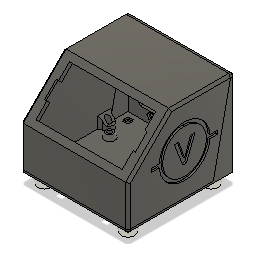
Voltímetro v10 (Autodesk Fusion 360 design; units mm, degrees)
Autodesk Fusion 360 part; units mm, degrees
note: some values were not read from the file. Set by a fixed rule: which face or edge a step refers to.
sketch "Sketch3" plane through (0, 0, 0) normal (0, 1, 0) x (1, 0, 0)
  circle A0 centre (-30.465, -17.5) radius 1.03 construction
  circle A1 centre (24.465, -17.5) radius 1.03 construction
  circle A2 centre (-30.465, 17.5) radius 1.03 construction
  circle A3 centre (24.465, 17.5) radius 1.03 construction
  line L0 (-30.465, 17.5) -> (24.465, 17.5) construction
  line L1 (24.465, 17.5) -> (24.465, -17.5) construction
  line L2 (24.465, -17.5) -> (-30.465, -17.5) construction
  line L3 (-30.465, -17.5) -> (-30.465, 17.5) construction
  line L4 (-30.465, 0) -> (24.465, 0) construction
  line L5 (-3, 17.5) -> (-3, -17.5) construction
  line L6 (-45, -42.5) -> (45, -42.5)
  line L7 (45, -42.5) -> (45, 47.5)
  line L8 (45, 47.5) -> (-45, 47.5)
  line L9 (-45, 47.5) -> (-45, -42.5)
  line L10 (0, -42.5) -> (0, 47.5) construction
  line L11 (-45, 44) -> (45, 44)
  circle A4 centre (-30.465, 17.5) radius 1.75
  circle A5 centre (-30.465, -17.5) radius 1.75
  circle A6 centre (24.465, -17.5) radius 1.75
  circle A7 centre (24.465, 17.5) radius 1.75
  circle A8 centre (-30.465, 17.5) radius 3.07
  circle A9 centre (-30.465, -17.5) radius 3.07
  circle A10 centre (24.465, -17.5) radius 3.07
  circle A11 centre (24.465, 17.5) radius 3.07
  dimension "d3" = 35
  dimension "d4" = 35
  dimension "d5" = 54.93
  dimension "d6" = 54.93
  dimension "d8" = 2.06
  dimension "d9" = 2.06
  dimension "d10" = 2.06
  dimension "d11" = 2.06
  dimension "d12" = 25
  dimension "d13" = 90
  dimension "d15" = 30
  dimension "d23" = 3.5
  dimension "d67" = 3.5
  dimension "d68" = 3.5
  dimension "d69" = 3.5
  dimension "d70" = 3.5
  dimension "d71" = 1.32
  dimension "d72" = 1.32
  dimension "d73" = 1.32
  dimension "d74" = 1.32
  dimension "d161" = 3
  constraint coincident A2.centre L0.start
  constraint coincident A3.centre L0.end
  constraint coincident A1.centre L1.end
  constraint coincident A0.centre L2.end
  constraint horizontal L0
  constraint vertical L3
  constraint midpoint L3 L4.start
  constraint midpoint L1 L4.end
  constraint midpoint L0 L5.start
  constraint midpoint L2 L5.end
  constraint horizontal L6
  constraint vertical L7
  constraint horizontal L8
  constraint vertical L9
  constraint midpoint L6 L10.start
  constraint midpoint L8 L10.end
  constraint coincident origin L10
  constraint coincident origin L4
  constraint coincident L9 L11.start
  constraint coincident L7 L11.end
  constraint perpendicular L7 L11
  constraint concentric A0 A5
  constraint concentric A1 A6
  constraint concentric A3 A7
  measures "d3" vertical distance of A0.centre A2.centre
  measures "d4" vertical distance of A1.centre A3.centre
  measures "d5" horizontal distance of A0.centre A1.centre
  measures "d6" horizontal distance of A2.centre A3.centre
  measures "d8" diameter of A2
  measures "d9" diameter of A3
  measures "d10" diameter of A1
  measures "d11" diameter of A0
  measures "d12" distance of L2 L6
  measures "d13" distance of L7 L9
  measures "d15" distance of L0 L8
  measures "d23" distance of L8 L11
  measures "d67" diameter of A4
  measures "d68" diameter of A5
  measures "d69" diameter of A6
  measures "d70" diameter of A7
  measures "d161" distance of L5 L10
extrude "Extrude1" add sketch "Sketch3" against normal blind 3.5 contours L6 L7 L9 L11 | L7 L8 L9 L11 | A4 | A5 | A6 | A7 | A8 | A9 | A10 | A11 makes body 1
sketch "Sketch4" plane through (0, 0, 0) normal (1, 0, 0) x (0, 0, -1)
  line L0 (-29.1643, 58.8035) -> (-68.5643, 58.8035)
  line L1 (-68.5643, 58.8035) -> (-68.5643, 33.8035)
  line L2 (-68.5643, 33.8035) -> (-29.1643, 33.8035)
  line L3 (-29.1643, 33.8035) -> (-29.1643, 58.8035)
  dimension "d19" = 25
  dimension "d20" = 39.4
  constraint horizontal L0
  constraint vertical L1
  constraint horizontal L2
  constraint vertical L3
  measures "d19" distance of L0 L2
  measures "d20" distance of L1 L3
extrude "Extrude2" add sketch "Sketch4" along normal mid plane 72 separate body makes body 2
move_body "Move1" bodies 2 to x (1, 0, 0) y (0, 0.707107, 0.707107) z (0, -0.707107, 0.707107) at (0, 49.8005, -24.0063)
extrude "Extrude3" add sketch "Sketch3" along normal blind 70 contours L7 L8 L9 L11 bodies 1
sketch "Sketch5" plane through (45, 0, 0) normal (1, 0, 0) x (0, 0, -1)
  line L0 (-42.5, 0) -> (47.5, 0)
  line L1 (44, 70) -> (29.121, 0)
  line L2 (44, 70) -> (135.3221, 70) construction
  line L3 (44, 0) -> (44, 70)
  point P0 (44, 70)
  dimension "d26" = 102
  constraint horizontal L2
  constraint coincident P0 L1.start
  constraint coincident L0 L1.end
  measures "d26" angle of L1 L2
extrude "Extrude4" add sketch "Sketch5" against normal blind 3.5 bodies 1
extrude "Extrude5" add sketch "Sketch5" along normal blind 3.5 from surface at -90 bodies 1
extrude "Extrude6" add sketch "Sketch3" along normal blind 70 separate body contours L6 L7 L9 L11 | L7 L8 L9 L11 | A4 | A5 | A6 | A7 | A8 | A9 | A10 | A11 makes body 3
chamfer "Chamfer1" distance 36 angle 45 1 edges at (0, 70, 42.5) on bodies 3
move_body "Move2" bodies 2 to x (1, 0, 0) y (0, 1, 0) z (0, 0, 1) at (0, 1.9818, -4.5415)
shell "Shell1" thickness 3.5 removed faces 1 at (-15, 0, 12.5) on bodies 3
combine "Combine1" operation cut target body 3 tool bodies 1 keep tools
sketch "Sketch6" plane through (0, 38.25, 38.25) normal (0, 0.707107, 0.707107) x (1, 0, 0)
  line L0 (45, -6.0104) -> (45, 44.9013)
  line L1 (45, 44.9013) -> (-45, 44.9013)
  line L2 (-45, 44.9013) -> (-45, -6.0104)
  line L3 (-45, -6.0104) -> (45, -6.0104)
  line L4 (-45, 19.4454) -> (45, 19.4454) construction
  line L5 (0, 44.9013) -> (0, -6.0104) construction
  line L6 (-36.2, 39.3454) -> (36.2, 39.3454)
  line L7 (36.2, 39.3454) -> (36.2, -0.4546)
  line L8 (36.2, -0.4546) -> (-36.2, -0.4546)
  line L9 (-36.2, -0.4546) -> (-36.2, 39.3454)
  line L10 (-36.2, 39.3454) -> (36.2, -0.4546) construction
  line L11 (36.2, 39.3454) -> (-36.2, -0.4546) construction
  point P0 (0, 19.4454)
  dimension "d151" = 2
  constraint midpoint L2 L4.start
  constraint midpoint L0 L4.end
  constraint midpoint L1 L5.start
  constraint midpoint L3 L5.end
  constraint horizontal L6
  constraint perpendicular L6 L7
  constraint parallel L6 L8
  constraint parallel L7 L9
  constraint coincident L10 P0
  constraint coincident L11 P0
  constraint midpoint L5 P0
  measures "d36" distance of L7.end L8.end
  measures "d37" distance of L6.end L7.end
extrude "Extrude7" cut sketch "Sketch6" against normal blind 10 contours L6 L7 L8 L9 bodies 3
sketch "Sketch7" plane through (0, 0, -47.5) normal (0, 0, -1) x (-1, 0, 0)
  line L0 (8.8, 56.65) -> (36, 56.65) construction
  line L1 (36, 56.65) -> (36, 15.1533) construction
  line L2 (30.6967, 9.85) -> (14.1033, 9.85) construction
  line L3 (8.8, 15.1533) -> (8.8, 56.65) construction
  line L4 (14.1033, 9.85) -> (8.8, 15.1533) construction
  line L5 (36, 15.1533) -> (30.6967, 9.85) construction
  line L6 (22.4, 56.65) -> (22.4, 9.85) construction
  line L7 (22.4, 33.25) -> (8.8, 33.25) construction
  circle A0 centre (22.4, 60.75) radius 1.75
  circle A1 centre (22.4, 5.75) radius 1.75
  line L8 (36.5, 57.15) -> (36.5, 14.9462)
  line L9 (36.5, 14.9462) -> (30.9038, 9.35)
  line L10 (30.9038, 9.35) -> (13.8962, 9.35)
  line L11 (13.8962, 9.35) -> (8.3, 14.9462)
  line L12 (8.3, 14.9462) -> (8.3, 57.15)
  line L13 (8.3, 57.15) -> (36.5, 57.15)
  line L14 (-45, 70) -> (-45, -3.5) construction
  line L15 (-45, -3.5) -> (45, -3.5) construction
  line L16 (45, -3.5) -> (45, 70) construction
  line L17 (45, 70) -> (-45, 70) construction
  line L18 (45, 33.25) -> (36.5, 33.25) construction
  line L19 (37.7, 58.35) -> (37.7, 14.4491) construction
  line L20 (37.7, 14.4491) -> (31.4009, 8.15) construction
  line L21 (31.4009, 8.15) -> (13.3991, 8.15) construction
  line L22 (13.3991, 8.15) -> (7.1, 14.4491) construction
  line L23 (7.1, 14.4491) -> (7.1, 58.35) construction
  line L24 (7.1, 58.35) -> (37.7, 58.35) construction
  point P0 (36, 9.85)
  point P1 (8.8, 9.85)
  dimension "d40" = 27.2
  dimension "d41" = 46.8
  dimension "d42" = 5.3033
  dimension "d43" = 5.3033
  dimension "d44" = 5.3033
  dimension "d45" = 5.3033
  dimension "d47" = 3.5
  dimension "d48" = 55
  dimension "d49" = -0.5
  dimension "d53" = 8.5
  dimension "d61" = -1.7
  constraint horizontal L0
  constraint vertical L1
  constraint horizontal L2
  constraint vertical L3
  constraint coincident P1 L2
  constraint coincident P1 L3
  constraint coincident P0 L1
  constraint coincident P0 L2
  constraint midpoint L0 L6.start
  constraint midpoint L2 L6.end
  constraint midpoint L6 L7.start
  constraint coincident L3 L7.end
  constraint perpendicular L3 L7
  constraint coincident L6 A0.centre
  constraint symmetric L7 A0 A1
  constraint midpoint L16 L18.start
  constraint perpendicular L16 L18
  constraint collinear L7 L18
  constraint coincident L8 L18.end
  measures "d40" distance of L0.start L0.end
  measures "d41" distance of L0.start P1
  measures "d42" distance of P1 L2.end
  measures "d43" distance of P1 L3.start
  measures "d44" distance of P0 L1.end
  measures "d45" distance of P0 L2.start
  measures "d47" diameter of A0
  measures "d48" distance of A0.centre A1.centre
  measures "d53" distance of L18.start L18.end
sketch "Sketch8" plane through (0, 0, -47.5) normal (0, 0, -1) x (-1, 0, 0)
  line L0 (-45, 70) -> (-45, -3.5)
  line L1 (-45, -3.5) -> (45, -3.5)
  line L2 (45, -3.5) -> (45, 70)
  line L3 (45, 70) -> (-45, 70)
  line L4 (-45, 33.25) -> (45, 33.25) construction
  circle A0 centre (-27.8532, 33.2847) radius 4.25
  line L5 (-27.8532, 33.2847) -> (-6.5468, 33.2847) construction
  circle A1 centre (-6.5468, 33.2847) radius 4.25
  line L6 (-17.2, 33.2847) -> (-17.2, 33.2153)
  circle A2 centre (-6.5468, 33.2847) radius 5 construction
  circle A3 centre (-27.8532, 33.2847) radius 5 construction
  line L7 (-41.5, 70) -> (-41.5, -3.5) construction
  line L8 (-45, 70) -> (-45, -3.5) construction
  line L9 (-27.8532, 33.2847) -> (-27.8532, 38.2847) construction
  line L10 (-27.8532, 38.2847) -> (-30.0921, 36.8972)
  line L11 (-27.8532, 38.2847) -> (-25.6144, 36.8972)
  line L12 (-6.5468, 33.2847) -> (-6.5468, 38.2847) construction
  line L13 (-6.5468, 38.2847) -> (-8.7856, 36.8972)
  line L14 (-6.5468, 38.2847) -> (-4.3079, 36.8972)
  line L15 (7.1, 14.4491) -> (7.1, 58.35)
  line L16 (7.1, 33.2625) -> (-41.5, 33.2625)
  point P0 (-17.2, 33.25)
  point P1 (-17.2, 33.2625)
  dimension "d54" = 8.5
  dimension "d55" = 8.5
  dimension "d57" = 10
  dimension "d58" = 10
  dimension "d59" = 3.5
  constraint midpoint L0 L4.start
  constraint midpoint L2 L4.end
  constraint coincident A0.centre L5.start
  constraint horizontal L5
  constraint coincident L5.end A1.centre
  constraint midpoint L5 L6.start
  constraint perpendicular L5 L6
  constraint concentric A1 A2
  constraint coincident L3 L7.start
  constraint coincident L1 L7.end
  constraint perpendicular L1 L7
  constraint midpoint L6 P0
  constraint coincident L4 P0
  constraint perpendicular L5 L9
  constraint coincident A3 L9.end
  constraint coincident A0 L10.end
  constraint tangent A0 L10
  constraint coincident A0 L11.end
  constraint tangent A0 L11
  constraint coincident A2 L12.end
  constraint perpendicular L5 L12
  constraint coincident A1 L13.end
  constraint tangent A1 L13
  constraint coincident A1 L14.end
  constraint tangent A1 L14
  constraint coincident L15 L16.start
  constraint coincident L7 L16.end
  constraint perpendicular L7 L16
  constraint midpoint L16 P1
  constraint coincident L6 P1
  measures "d54" diameter of A0
  measures "d55" diameter of A1
  measures "d57" diameter of A2
  measures "d58" diameter of A3
  measures "d59" distance of L7 L8
extrude "Extrude8" cut sketch "Sketch7" sketch "Sketch8" against normal blind 13.966 of sketch 2 contours A0 L16 | A0 L16 | A0 L10 L11 | A1 L16 | A1 L16 | A1 L13 L14 bodies 1
sketch "Sketch9" plane through (0, 0, -44) normal (0, 0, 1) x (1, 0, 0)
  circle A0 centre (-22.4, 5.75) radius 1.75
  circle A1 centre (-22.4, 60.75) radius 1.75
  line L0 (-24.0108, 8.54) -> (-25.6216, 5.75)
  line L1 (-25.6216, 5.75) -> (-24.0108, 2.96)
  line L2 (-24.0108, 2.96) -> (-20.7892, 2.96)
  line L3 (-20.7892, 2.96) -> (-19.1784, 5.75)
  line L4 (-19.1784, 5.75) -> (-20.7892, 8.54)
  line L5 (-20.7892, 8.54) -> (-24.0108, 8.54)
  line L6 (-24.0108, 63.54) -> (-25.6216, 60.75)
  line L7 (-25.6216, 60.75) -> (-24.0108, 57.96)
  line L8 (-24.0108, 57.96) -> (-20.7892, 57.96)
  line L9 (-20.7892, 57.96) -> (-19.1784, 60.75)
  line L10 (-19.1784, 60.75) -> (-20.7892, 63.54)
  line L11 (-20.7892, 63.54) -> (-24.0108, 63.54)
  point P0 (-22.4, 60.75)
  point P1 (-22.4, 5.75)
  point P2 (-22.4, 5.75)
  point P3 (-22.4, 60.75)
  dimension "d103" = 2.79
  dimension "d104" = 2.79
  constraint coincident P0 A1.centre
  constraint coincident P2 A0.centre
  constraint coincident P2 P1
  constraint horizontal L5
  constraint horizontal L11
  measures "d103" distance of P2 L5
  measures "d104" distance of P3 L11
extrude "Extrude9" cut sketch "Sketch9" against normal blind 1.5 contours A1 | L0 L1 L2 L3 L4 L5 | L6 L7 L8 L9 L10 L11 bodies 1
extrude "Extrude10" add sketch "Sketch3" along normal blind 4 contours A8 | A9 | A10 | A11 bodies 1
chamfer "Chamfer2" distance 1.45 angle 70 4 edges at (-33.3272, 0, 16.3898) (-33.3272, 0, -18.6102) (21.6028, 0, -18.6102) (21.6028, 0, 16.3898) measured on face at (5.3095, 0, 5.2569) measured on face at (5.3095, 0, 5.2569) measured on face at (5.3095, 0, 5.2569) measured on face at (5.3095, 0, 5.2569) on bodies 1
move_body "Move3" bodies 2 to x (1, 0, 0) y (0, 1, 0) z (0, 0, 1) at (0, -2.111, -23.1451)
move_body "Move4" bodies 2 to x (1, 0, 0) y (0, 1, 0) z (0, 0, 1) at (0, -1.9366, 2.7021)
sketch "Sketch10" plane through (0, -3.5, 0) normal (0, -1, 0) x (1, 0, 0)
  line L0 (-45, 42.5) -> (-45, -47.5)
  line L1 (-45, -47.5) -> (45, -47.5)
  line L2 (45, -47.5) -> (45, 42.5)
  line L3 (45, 42.5) -> (-45, 42.5)
  circle A0 centre (-35, 32.5) radius 7.5
  line L4 (-45, -2.5) -> (45, -2.5) construction
  line L5 (0, 42.5) -> (0, -47.5) construction
  circle A1 centre (35, 32.5) radius 7.5
  circle A2 centre (-35, -37.5) radius 7.5
  circle A3 centre (35, -37.5) radius 7.5
  circle A4 centre (-35, 32.5) radius 1.75
  circle A5 centre (35, 32.5) radius 1.75
  circle A6 centre (-35, -37.5) radius 1.75
  circle A7 centre (35, -37.5) radius 1.75
  line L6 (-36.6108, 35.29) -> (-38.2216, 32.5)
  line L7 (-38.2216, 32.5) -> (-36.6108, 29.71)
  line L8 (-36.6108, 29.71) -> (-33.3892, 29.71)
  line L9 (-33.3892, 29.71) -> (-31.7784, 32.5)
  line L10 (-31.7784, 32.5) -> (-33.3892, 35.29)
  line L11 (-33.3892, 35.29) -> (-36.6108, 35.29)
  line L12 (38.2216, 32.5) -> (36.6108, 29.71)
  line L13 (36.6108, 29.71) -> (33.3892, 29.71)
  line L14 (33.3892, 29.71) -> (31.7784, 32.5)
  line L15 (31.7784, 32.5) -> (33.3892, 35.29)
  line L16 (33.3892, 35.29) -> (36.6108, 35.29)
  line L17 (36.6108, 35.29) -> (38.2216, 32.5)
  line L18 (-31.7784, -37.5) -> (-33.3892, -40.29)
  line L19 (-33.3892, -40.29) -> (-36.6108, -40.29)
  line L20 (-36.6108, -40.29) -> (-38.2216, -37.5)
  line L21 (-38.2216, -37.5) -> (-36.6108, -34.71)
  line L22 (-33.3892, -34.71) -> (-31.7784, -37.5)
  line L23 (-36.6108, -34.71) -> (-33.3892, -34.71)
  line L24 (36.6108, -40.29) -> (38.2216, -37.5)
  line L25 (38.2216, -37.5) -> (36.6108, -34.71)
  line L26 (36.6108, -34.71) -> (33.3892, -34.71)
  line L27 (33.3892, -34.71) -> (31.7784, -37.5)
  line L28 (33.3892, -40.29) -> (36.6108, -40.29)
  line L29 (31.7784, -37.5) -> (33.3892, -40.29)
  point P0 (-35, 32.5)
  dimension "d80" = 15
  dimension "d81" = 10
  dimension "d82" = 10
  dimension "d91" = 3.5
  dimension "d92" = 3.5
  dimension "d93" = 3.5
  dimension "d94" = 3.5
  dimension "d95" = 2.79
  constraint midpoint L0 L4.start
  constraint midpoint L2 L4.end
  constraint midpoint L3 L5.start
  constraint midpoint L1 L5.end
  constraint symmetric A0 L5 A1
  constraint symmetric A0 L4 A2
  constraint symmetric L4 A1 A3
  constraint concentric A0 A4
  constraint concentric A1 A5
  constraint concentric A2 A6
  constraint concentric A3 A7
  constraint coincident P0 A0.centre
  constraint symmetric L5 L6.start L16.end
  constraint symmetric L5 L6.end L12.start
  constraint symmetric L5 L7.end L12.end
  constraint symmetric L5 L8.end L13.end
  constraint symmetric L5 L9.end L14.end
  constraint symmetric L5 L10.end L15.end
  constraint symmetric L4 L6.start L19.end
  constraint symmetric L4 L6.end L20.end
  constraint symmetric L4 L7.end L21.end
  constraint symmetric L4 L8.end L22.start
  constraint symmetric L4 L9.end L18.start
  constraint symmetric L4 L10.end L18.end
  constraint symmetric L4 L12.start L24.end
  constraint symmetric L4 L12.end L25.end
  constraint symmetric L4 L13.end L26.end
  constraint symmetric L4 L14.end L27.end
  constraint symmetric L4 L15.end L28.start
  constraint symmetric L4 L16.end L24.start
  constraint horizontal L11
  measures "d80" diameter of A0
  measures "d81" distance of L0 P0
  measures "d82" distance of L3 P0
  measures "d91" diameter of A4
  measures "d92" diameter of A5
  measures "d93" diameter of A6
  measures "d94" diameter of A7
  measures "d95" distance of P0 L11
extrude "Extrude11" add sketch "Sketch10" along normal blind 7.5 draft -15 separate body contours A0 | A4 | L6 L7 L8 L9 L10 L11 makes body 4
sketch "Sketch11" plane through (0, -11, 0) normal (0, -1, 0) x (1, 0, 0)
  circle A0 centre (-35, 32.5) radius 5.4904
  circle A1 centre (-35, 32.5) radius 3.625
  circle A2 centre (-35, 32.5) radius 1.55
  dimension "d85" = 7.25
  dimension "d86" = 3.1
  constraint concentric A0 A1
  constraint concentric A0 A2
  measures "d85" diameter of A1
  measures "d86" diameter of A2
extrude "Extrude12" cut sketch "Sketch11" against normal blind 5 contours A1 bodies 4
extrude "Extrude13" cut sketch "Sketch11" against normal blind 20.575 contours A2 bodies 4
extrude "Extrude14" cut sketch "Sketch10" along normal blind 1.5 from surface at -3.5 contours L6 L7 L8 L9 L10 L11 | L12 L13 L14 L15 L16 L17 | L18 L19 L20 L21 L22 L23 | L24 L25 L26 L27 L28 L29 bodies 1
extrude "Extrude15" cut sketch "Sketch10" against normal blind 7.44 contours A4 | A5 | A6 | A7 bodies 1
sketch "Sketch12" plane through (0, 0, 0) normal (0, 1, 0) x (-1, 0, 0)
  line L0 (-36.6108, 35.29) -> (-33.3892, 35.29)
  line L1 (-33.3892, 35.29) -> (-31.7784, 32.5)
  line L2 (-31.7784, 32.5) -> (-33.3892, 29.71)
  line L3 (-33.3892, 29.71) -> (-36.6108, 29.71)
  line L4 (-36.6108, 29.71) -> (-38.2216, 32.5)
  line L5 (-38.2216, 32.5) -> (-36.6108, 35.29)
  line L6 (36.6108, -34.71) -> (38.2216, -37.5)
  line L7 (38.2216, -37.5) -> (36.6108, -40.29)
  line L8 (36.6108, -40.29) -> (33.3892, -40.29)
  line L9 (33.3892, -40.29) -> (31.7784, -37.5)
  line L10 (31.7784, -37.5) -> (33.3892, -34.71)
  line L11 (33.3892, -34.71) -> (36.6108, -34.71)
  line L12 (33.3892, 35.29) -> (36.6108, 35.29)
  line L13 (36.6108, 35.29) -> (38.2216, 32.5)
  line L14 (38.2216, 32.5) -> (36.6108, 29.71)
  line L15 (36.6108, 29.71) -> (33.3892, 29.71)
  line L16 (33.3892, 29.71) -> (31.7784, 32.5)
  line L17 (31.7784, 32.5) -> (33.3892, 35.29)
  line L18 (-31.7784, -37.5) -> (-33.3892, -40.29)
  line L19 (-33.3892, -40.29) -> (-36.6108, -40.29)
  line L20 (-36.6108, -40.29) -> (-38.2216, -37.5)
  line L21 (-38.2216, -37.5) -> (-36.6108, -34.71)
  line L22 (-36.6108, -34.71) -> (-33.3892, -34.71)
  line L23 (-33.3892, -34.71) -> (-31.7784, -37.5)
  line L24 (41.5, -29.121) -> (45, -29.121)
  line L25 (45, -29.121) -> (45, 42.5)
  line L26 (45, 42.5) -> (-45, 42.5)
  line L27 (-45, 42.5) -> (-45, -29.121)
  line L28 (-45, -29.121) -> (-41.5, -29.121)
  line L29 (-41.5, -29.121) -> (-41.5, -44)
  line L30 (-41.5, -44) -> (41.5, -44)
  line L31 (41.5, -44) -> (41.5, -29.121)
  line L32 (0, -44) -> (0, 42.5) construction
  circle A0 centre (38, -23.971) radius 2.25
  circle A1 centre (38, -23.971) radius 4.32
  circle A2 centre (-38, -23.971) radius 4.32
  circle A3 centre (-38, -23.971) radius 2.25
  circle A4 centre (19, 35.5) radius 4.32
  circle A5 centre (19, 35.5) radius 2.25
  circle A6 centre (-19, 35.5) radius 4.32
  circle A7 centre (-19, 35.5) radius 2.25
  circle A8 centre (19, 35.5) radius 1.75
  circle A9 centre (-19, 35.5) radius 1.75
  circle A10 centre (38, -23.971) radius 1.75
  circle A11 centre (-38, -23.971) radius 1.75
  circle A12 centre (-24.465, -17.5) radius 4.52
  circle A13 centre (30.465, 17.5) radius 4.52
  circle A14 centre (30.465, -17.5) radius 4.52
  circle A15 centre (-24.465, 17.5) radius 4.52
  dimension "d105" = 4.5
  dimension "d106" = 2.07
  dimension "d107" = 7
  dimension "d108" = 5.15
  dimension "d109" = 2.07
  dimension "d110" = 4.5
  dimension "d111" = 7
  dimension "d112" = 19
  dimension "d113" = 3.5
  dimension "d114" = 3.5
  constraint midpoint L30 L32.start
  constraint midpoint L26 L32.end
  constraint symmetric L32 A0 A3
  constraint symmetric L32 A1 A2
  constraint symmetric L32 A4 A6
  constraint symmetric L32 A5 A7
  constraint concentric A5 A8
  constraint symmetric L32 A8 A9
  constraint concentric A0 A10
  constraint symmetric L32 A10 A11
  measures "d105" diameter of A0
  measures "d107" distance of L25 A0.centre
  measures "d108" vertical distance of L24.start A0.centre
  measures "d110" diameter of A5
  measures "d111" distance of L26 A4.centre
  measures "d112" distance of L32 A4.centre
  measures "d113" diameter of A8
  measures "d114" diameter of A10
extrude "Extrude16" cut sketch "Sketch12" against normal blind 8.444 contours A8 | A9 | A10 | A11 bodies 1
sketch "Sketch13" plane through (0, -3.5, 0) normal (0, -1, 0) x (1, 0, 0)
  circle A0 centre (-19, 35.5) radius 1.75
  circle A1 centre (19, 35.5) radius 1.75
  circle A2 centre (38, -23.971) radius 1.75
  circle A3 centre (-38, -23.971) radius 1.75
  circle A4 centre (-38, -23.971) radius 3.75
  circle A5 centre (-19, 35.5) radius 3.75
  circle A6 centre (19, 35.5) radius 3.75
  circle A7 centre (38, -23.971) radius 3.75
  dimension "d117" = 7.5
  dimension "d118" = 7.5
  dimension "d119" = 7.5
  dimension "d120" = 7.5
  constraint concentric A3 A4
  constraint concentric A0 A5
  constraint concentric A1 A6
  constraint concentric A2 A7
  measures "d117" diameter of A4
  measures "d118" diameter of A5
  measures "d119" diameter of A6
  measures "d120" diameter of A7
extrude "Extrude17" cut sketch "Sketch13" against normal blind 1.5 bodies 1
extrude "Extrude18" add sketch "Sketch12" along normal blind 4 contours A0 | A1 | A2 | A3 | A4 | A5 | A6 | A7 | A8 | A9 | A10 | A11 bodies 3
sketch "Sketch14" plane through (0, 0, -44) normal (0, 0, 1) x (1, 0, 0)
  circle A0 centre (0, 63) radius 4.89
  circle A1 centre (0, 63) radius 2.25
  circle A2 centre (0, 63) radius 1.75
  line L0 (-41.5, 70) -> (41.5, 70)
  line L1 (0, 70) -> (0, 55.075) construction
  line L2 (41.5, 66.5) -> (-41.5, 66.5)
  line L3 (4.89, 63) -> (-4.89, 63) construction
  line L4 (4.89, 63) -> (4.89, 66.5)
  line L5 (-4.89, 63) -> (-4.89, 66.5)
  dimension "d125" = 2.64
  dimension "d126" = 4.5
  dimension "d127" = 3.5
  dimension "d158" = 7
  constraint concentric A1 A2
  constraint midpoint L0 L1.start
  constraint perpendicular L0 L1
  constraint coincident A0.centre A1.centre
  constraint coincident A0 L3.start
  constraint coincident A0 L3.end
  constraint horizontal L3
  constraint coincident L2 L4.end
  constraint tangent A0 L4
  constraint perpendicular L2 L4
  constraint coincident L2 L5.end
  constraint tangent A0 L5
  measures "d126" diameter of A1
  measures "d127" diameter of A2
  measures "d158" distance of A0.centre L0
extrude "Extrude19" cut sketch "Sketch14" against normal blind 9.767 contours A2 bodies 1
extrude "Extrude20" add sketch "Sketch14" along normal blind 4 contours A0 L2 | A0 L2 | A1 | A2 bodies 3
chamfer "Chamfer3" distance 5.524 angle 45 5 edges at (0, 66.5, -40) (19, 4, 39) (-19, 4, 39) (41.5, 4, -23.971) (-41.5, 4, -23.971) measured on face at (1.1383, 66.5, -9.9665) measured on face at (5.4892, 23.0335, 39) measured on face at (5.4892, 23.0335, 39) measured on face at (41.5, 45.6667, -19.8815) measured on face at (-41.5, 45.6667, -19.8815) on bodies 3
extrude "Extrude21" cut sketch "Sketch12" along normal blind 9.55 contours A0 | A3 | A5 | A7 | A8 | A9 | A10 | A11 bodies 3
extrude "Extrude22" cut sketch "Sketch14" along normal blind 9.55 contours A1 | A2 bodies 3
sketch "Sketch15" plane through (0, 0, -47.5) normal (0, 0, -1) x (-1, 0, 0)
  circle A0 centre (0, 63) radius 1.75
  circle A1 centre (0, 63) radius 3.75
  dimension "d138" = 7.5
  constraint concentric A0 A1
  measures "d138" diameter of A1
extrude "Extrude23" cut sketch "Sketch15" against normal blind 1.5 bodies 1
sketch "Sketch16" plane through (0, 38.25, 38.25) normal (0, 0.707107, 0.707107) x (1, 0, 0)
  line L0 (-36.2, -0.4546) -> (-36.2, 39.3454)
  line L1 (-36.2, 39.3454) -> (36.2, 39.3454)
  line L2 (36.2, 39.3454) -> (36.2, -0.4546)
  line L3 (36.2, -0.4546) -> (-36.2, -0.4546)
  line L4 (-36.2, 19.4454) -> (36.2, 19.4454) construction
  line L5 (-39.6, 26.4454) -> (-36.2, 26.4454)
  line L6 (-36.2, 26.4454) -> (-36.2, 12.4454)
  line L7 (-36.2, 12.4454) -> (-39.6, 12.4454)
  line L8 (-39.6, 12.4454) -> (-39.6, 26.4454)
  line L9 (-36.2, 19.4454) -> (-39.6, 19.4454) construction
  line L10 (0, 39.3454) -> (0, -0.4546) construction
  line L11 (36.2, 26.4454) -> (36.2, 12.4454)
  line L12 (36.2, 12.4454) -> (39.6, 12.4454)
  line L13 (39.6, 12.4454) -> (39.6, 26.4454)
  line L14 (39.6, 26.4454) -> (36.2, 26.4454)
  line L15 (38.15, 26.4454) -> (38.15, 12.4454)
  line L16 (-38.15, 26.4454) -> (-38.15, 12.4454)
  dimension "d141" = 3.4
  dimension "d142" = 14
  dimension "d153" = 1.95
  dimension "d154" = 1.95
  constraint midpoint L0 L4.start
  constraint midpoint L2 L4.end
  constraint horizontal L5
  constraint vertical L6
  constraint horizontal L7
  constraint vertical L8
  constraint midpoint L4.start L6
  constraint midpoint L8 L9.end
  constraint midpoint L1 L10.start
  constraint midpoint L3 L10.end
  constraint symmetric L5.start L10 L13.end
  constraint symmetric L5.end L10 L11.start
  constraint symmetric L6.end L10 L11.end
  constraint symmetric L7.end L10 L12.end
  constraint coincident L14 L15.start
  constraint coincident L12 L15.end
  constraint perpendicular L12 L15
  constraint coincident L5 L16.start
  constraint coincident L7 L16.end
  constraint perpendicular L7 L16
  measures "d141" distance of L5.start L5.end
  measures "d142" distance of L5.start L7.end
  measures "d153" distance of L11 L15
  measures "d154" distance of L6 L16
extrude "Extrude24" cut sketch "Sketch16" against normal up to surface (1.5 mm away) from surface at -2 contours L0 L5 L6 L7 L16 | L5 L7 L8 L16 | L2 L11 L12 L14 L15 | L12 L13 L14 L15 bodies 3
pattern_linear "R-Pattern1" count 2 spacing 70 along (0, 0, -1) count 2 spacing 70 along (1, 0, 0) of bodies 4 makes body 5 at (-28.6451, -5.1667, -34.4396) makes body 6 at (41.3549, -5.1667, 35.5604) makes body 7 at (41.3549, -5.1667, -34.4396)
move_body "Move5" bodies 2 to x (1, 0, 0) y (0, 1, 0) z (0, 0, 1) at (0, -2.2804, -2.1409)
chamfer "Chamfer4" distance 2 angle 45 17 edges at (45, -1.75, 42.5) (-45, -1.75, 42.5) (0, -3.5, 42.5) (45, -3.5, -2.5) (45, 33.25, -47.5) (-45, 33.25, -47.5) (-45, -3.5, -2.5) (0, -3.5, -47.5) (-45, 70, -45.75) (45, 70, -45.75) (0, 70, -47.5) (-45, 70, -18.75) (45, 70, -18.75) (45, 17, 42.5) (-45, 17, 42.5) (-45, 52, 24.5) (45, 52, 24.5) on bodies 1 3
extrude "Extrude25" cut sketch "Sketch16" against normal blind 6.007 contours L0 L5 L6 L7 L16 | L2 L11 L12 L14 L15 bodies 3
chamfer "Chamfer6" distance 1.5 angle 45 2 edges at (-8.3, 57.15, -45.75) (-36.5, 57.15, -45.75) on bodies 1
chamfer "Chamfer7" distance 3 angle 45 10 edges at (3.415, 66.5, -39.238) (-3.415, 66.5, -39.238) (41.5, 4.762, -26.5033) (41.5, 4.762, -21.4388) (-41.5, 4.762, -26.5033) (-41.5, 4.762, -21.4388) (-21.5323, 4.762, 39) (-16.4677, 4.762, 39) (16.4677, 4.762, 39) (21.5323, 4.762, 39) on bodies 3
ref_plane "WorkPlane3" through (24.465, 24, 17.5) normal (0, 1, 0) x (1, 0, 0)
sketch "Sketch17" plane through (0, 24, 0) normal (0, 1, 0) x (1, 0, 0)
  line L0 (-36, 6.6067) -> (36, 6.6067)
  line L1 (36, 6.6067) -> (36, -21.2533)
  line L2 (36, -21.2533) -> (-36, -21.2533)
  line L3 (-36, -21.2533) -> (-36, 6.6067)
  line L4 (36, -21.6072) -> (-36, -21.6072)
  circle A0 centre (24.465, -17.5) radius 1.75
  constraint coincident L1 L4.start
  constraint coincident L3 L4.end
  constraint perpendicular L3 L4
sketch "Sketch18" plane through (0, 0, -47.5) normal (0, 0, -1) x (-1, 0, 0)
  circle A0 centre (22.4, 5.75) radius 1.75
  circle A1 centre (22.4, 60.75) radius 1.75
  circle A2 centre (0, 63) radius 1.75
  circle A3 centre (0, 63) radius 2.1
  circle A4 centre (22.4, 60.75) radius 2.1
  circle A5 centre (22.4, 5.75) radius 2.1
  line L0 (22.4, 5.75) -> (22.4, 7.85)
  line L1 (22.4, 7.85) -> (21.4327, 7.2083)
  line L2 (22.4, 7.85) -> (23.3673, 7.2083)
  line L3 (22.4, 60.75) -> (22.4, 62.85)
  line L4 (22.4, 62.85) -> (21.4327, 62.2083)
  line L5 (22.4, 62.85) -> (23.3673, 62.2083)
  line L6 (0, 63) -> (0, 65.1)
  line L7 (0, 65.1) -> (-0.9673, 64.4583)
  line L8 (0, 65.1) -> (0.9673, 64.4583)
  circle A6 centre (0, 63) radius 3.75
  circle A7 centre (0, 63) radius 4.5
  line L9 (0, 63) -> (0, 67.5)
  line L10 (0, 67.5) -> (-2.0729, 66.125)
  line L11 (0, 67.5) -> (2.0729, 66.125)
  dimension "d162" = 0.35
  dimension "d163" = 0.35
  dimension "d164" = 0.35
  dimension "d167" = 0.75
  constraint coincident A0.centre A5.centre
  constraint coincident A5 L0.end
  constraint vertical L0
  constraint coincident A0 L1.end
  constraint tangent A0 L1
  constraint coincident A0 L2.end
  constraint tangent A0 L2
  constraint coincident A1.centre A4.centre
  constraint coincident A4 L3.end
  constraint parallel L0 L3
  constraint coincident A1 L4.end
  constraint tangent A1 L4
  constraint coincident A1 L5.end
  constraint tangent A1 L5
  constraint coincident A2.centre A3.centre
  constraint coincident A3 L6.end
  constraint parallel L3 L6
  constraint coincident A2 L7.end
  constraint tangent A2 L7
  constraint coincident A2 L8.end
  constraint tangent A2 L8
  constraint coincident A7 L9.end
  constraint parallel L6 L9
  constraint coincident A6 L10.end
  constraint tangent A6 L10
  constraint coincident A6 L11.end
  constraint tangent A6 L11
extrude "Extrude26" cut sketch "Sketch18" against normal blind 9.723 contours A0 L0 L2 | A0 L0 L1 | A1 | A1 L3 L5 | A1 L3 L4 | A2 | A2 L6 L8 L9 | A2 L6 L7 L9 bodies 1
extrude "Extrude27" cut sketch "Sketch18" against normal up to surface (1.5 mm away) contours A6 L9 L11 | A6 L9 L10 bodies 1
sketch "Sketch19" plane through (45, 0, 0) normal (1, 0, 0) x (0, 0, -1)
  line L0 (32.52, 35.3126) -> (26.2043, 35.3126)
  spline S0 degree 3 poles (26.2043, 35.3126) (25.4634, 46.3731) (16.2304, 55.1455) (4.9857, 55.1455) knots 0 0 0 0 1 1 1 1
  spline S1 degree 3 poles (4.9857, 55.1455) (-6.2591, 55.1455) (-15.4921, 46.3731) (-16.2329, 35.3126) knots 0 0 0 0 1 1 1 1
  line L1 (-16.2329, 35.3126) -> (-22.672, 35.3126)
  line L2 (-22.672, 35.3126) -> (-22.672, 32.3493)
  line L3 (-22.672, 32.3493) -> (-16.2272, 32.3493)
  spline S2 degree 3 poles (-16.2272, 32.3493) (-15.4411, 21.3325) (-6.2278, 12.609) (4.9857, 12.609) knots 0 0 0 0 1 1 1 1
  spline S3 degree 3 poles (4.9857, 12.609) (16.1991, 12.609) (25.4125, 21.3325) (26.1985, 32.3493) knots 0 0 0 0 1 1 1 1
  line L4 (26.1985, 32.3493) -> (32.52, 32.3493)
  line L5 (32.52, 32.3493) -> (32.52, 35.3126)
  spline S4 degree 3 poles (23.2906, 33.8772) (23.2906, 23.7839) (15.079, 15.5724) (4.9857, 15.5724) knots 0 0 0 0 1 1 1 1
  spline S5 degree 3 poles (4.9857, 15.5724) (-5.1076, 15.5724) (-13.3192, 23.7839) (-13.3192, 33.8772) knots 0 0 0 0 1 1 1 1
  spline S6 degree 3 poles (-13.3192, 33.8772) (-13.3192, 43.9705) (-5.1076, 52.1821) (4.9857, 52.1821) knots 0 0 0 0 1 1 1 1
  spline S7 degree 3 poles (4.9857, 52.1821) (15.079, 52.1821) (23.2906, 43.9705) (23.2906, 33.8772) knots 0 0 0 0 1 1 1 1
  line L6 (9.9406, 42.9061) -> (5.0372, 29.0476)
  line L7 (5.0372, 29.0476) -> (0.0821, 42.9061)
  line L8 (0.0821, 42.9061) -> (-3.66, 42.9061)
  line L9 (-3.66, 42.9061) -> (3.5403, 24.5705)
  line L10 (3.5403, 24.5705) -> (6.534, 24.5705)
  line L11 (6.534, 24.5705) -> (13.6827, 42.9061)
  line L12 (13.6827, 42.9061) -> (9.9406, 42.9061)
extrude "Extrude28" cut sketch "Sketch19" against normal blind 1.5 bodies 3
extrude "Extrude29" cut sketch "Sketch19" along normal blind 1.5 from surface at -90 bodies 3
hidden bodies 2
equation "d43 = d42"
equation "d45 = d44"
equation "d53 = 3.5 mm + 5 mm"
equation "d57 = d58"
equation "d71 = ( 0.6 * 1.1 * 2 ) * 1 mm"
equation "d72 = ( 0.6 * 1.1 * 2 ) * 1 mm"
equation "d73 = ( 0.6 * 1.1 * 2 ) * 1 mm"
equation "d74 = ( 0.6 * 1.1 * 2 ) * 1 mm"
equation "d95 = ( ( 5.33 + 0.25 ) / 2 ) * 1 mm"
equation "d103 = ( ( 5.33 + 0.25 ) / 2 ) * 1 mm"
equation "d104 = ( ( 5.33 + 0.25 ) / 2 ) * 1 mm"
equation "d106 = ( 0.6 * 1.15 * 3 ) * 1 mm"
equation "d109 = ( 0.6 * 1.15 * 3 ) * 1 mm"
equation "d125 = ( 0.6 * 1.1 * 4 ) * 1 mm"
named bodies: "Cuerpo", "Tapa"
